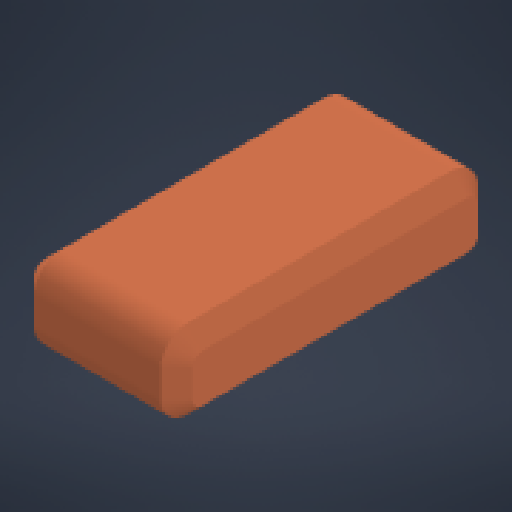
# Autodesk Inventor part: battery
Saved by Autodesk Inventor 2026.2 (Build 302298000, 298)
## iProperties
Created: 2025-07-12
Part Number: battery
Material: Generic
Document SubType Name: Modeling
Designer: micyg
Density: 1 g/cm^3
Appearance: Default
Author: micyg
Autodesk Inventor part; units mm, degrees
ref_plane "YZ Plane" through (0, 0, 0) normal (1, 0, 0) x (0, 1, 0)
ref_plane "XZ Plane" through (0, 0, 0) normal (0, 1, 0) x (-1, 0, 0)
ref_plane "XY Plane" through (0, 0, 0) normal (0, 0, 1) x (1, 0, 0)
sketch "Sketch1" plane through (0, 0, 0) normal (0, 1, 0) x (-1, 0, 0)
  line L0 (0, 0) -> (20, 0)
  line L1 (20, 0) -> (20, -40)
  line L2 (20, -40) -> (0, -40)
  line L3 (0, -40) -> (0, 0)
  dimension "d0" = 20
  dimension "d1" = 40
  constraints: 8 end point, 2 parallel, 1 horizontal, 1 perpendicular
  measures "d0" distance of L1.end L2.end
  measures "d1" distance of L0.end L1.end
extrude "Extrusion1" add sketch "Sketch1" along normal blind 10
fillet "Fillet1" radius 3.3333 4 edges at (-10, 10, 0) (-10, 0, 0) (-10, 10, -40) (-10, 0, -40)
chamfer "Chamfer1" distance 2 angle 45 8 edges at (0, 10, -20) (0, 9.0237, -39.0237) (0, 0, -20) (0, 9.0237, -0.9763) (-20, 10, -20) (-20, 9.0237, -0.9763) (-20, 0, -20) (-20, 9.0237, -39.0237)
equation "\"d4\" = 0.333333 * d2"
equation "\"d2\" = 10"
body "Solid1"
